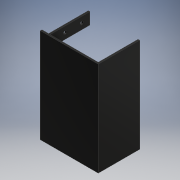
# Autodesk Inventor part: elbow servo plate
Saved by Autodesk Inventor 2017 (Build 210142000, 142)
## iProperties
Created: 2018-10-18
Part Number: elbow servo plate
Material: Generic
Document SubType Name: Modeling
Designer: Cameron
Density: 1 g/cm^3
Appearance: Glossy - Black
Author: Cameron
Autodesk Inventor part; units mm, degrees
ref_plane "YZ Plane" through (0, 0, 0) normal (1, 0, 0) x (0, 1, 0)
ref_plane "XZ Plane" through (0, 0, 0) normal (0, 1, 0) x (-1, 0, 0)
ref_plane "XY Plane" through (0, 0, 0) normal (0, 0, 1) x (1, 0, 0)
sketch "Sketch1" plane through (0, 0, 0) normal (0, 1, 0) x (-1, 0, 0)
  line L0 (0, 0) -> (35, 0)
  line L1 (35, 0) -> (35, -57)
  line L2 (35, -57) -> (0, -57)
  line L3 (0, -57) -> (0, 0)
  dimension "d0" = 35
  dimension "d1" = 57
  constraints: 8 end point, 2 parallel, 1 horizontal, 1 perpendicular
  measures "d0" distance of L1.end L2.end
  measures "d1" distance of L0.end L1.end
extrude "Extrusion1" add sketch "Sketch1" along normal blind 1
sketch "Sketch2" plane through (0, 1, 0) normal (0, 1, 0) x (1, 0, 0)
  line L0 (-35, 0) -> (0, 0) projected
  line L1 (0, 57) -> (-35, 57) projected
  line L2 (0, 0) -> (-1, 0)
  line L3 (-1, 0) -> (-1, 57)
  line L4 (-1, 57) -> (0, 57)
  line L5 (0, 57) -> (0, 0)
  line L6 (-31, 0) -> (-30, 0)
  line L7 (-30, 0) -> (-30, 7)
  line L8 (-30, 7) -> (-31, 7)
  line L9 (-31, 7) -> (-31, 0)
  line L10 (-31, 57) -> (-30, 57)
  line L11 (-30, 57) -> (-30, 50)
  line L12 (-30, 50) -> (-31, 50)
  line L13 (-31, 50) -> (-31, 57)
  dimension "d4" = 1
  dimension "d5" = 31
  dimension "d6" = 1
  dimension "d7" = 7
  dimension "d8" = 7
  constraints: 24 end point, 8 point on line, 5 perpendicular, 2 parallel, 1 horizontal
  measures "d4" distance of L3.end L4.end
  measures "d5" distance of L0.end L6.start
  measures "d6" distance of L6.start L6.end
  measures "d7" distance of L6.end L7.end
  measures "d8" distance of L10.end L11.end
extrude "Extrusion2" add sketch "Sketch2" along normal blind 24
sketch "Sketch3" plane through (-30, 1, 0) normal (1, 0, 0) x (0, 0, -1)
  line L0 (0, 24) -> (7, 24) projected
  line L1 (3.5, 24) -> (3.5, 19)
  line L2 (3.5, 19) -> (3.5, 9)
  line L3 (50, 24) -> (57, 24) projected
  line L4 (53.5, 24) -> (53.5, 19)
  line L5 (53.5, 19) -> (53.5, 9)
  circle A0 centre (3.5, 19) radius 1
  circle A1 centre (3.5, 9) radius 1
  circle A2 centre (53.5, 19) radius 1
  circle A3 centre (53.5, 9) radius 1
  point P0 (0, -1)
  dimension "d11" = 5
  dimension "d12" = 10
  dimension "d13" = 5
  dimension "d14" = 10
  dimension "d15" = 2
  dimension "d16" = 2
  dimension "d17" = 2
  dimension "d18" = 2
  constraints: 8 end point, 4 centre point, 4 coincident, 2 midpoint, 2 point on line, 2 vertical
  measures "d11" distance of L1.start L1.end
  measures "d12" distance of L1.end L2.end
  measures "d13" distance of L4.start L4.end
  measures "d14" distance of L4.end L5.end
  measures "d15" diameter of A0
  measures "d16" diameter of A1
  measures "d17" diameter of A2
  measures "d18" diameter of A3
extrude "Extrusion3" cut sketch "Sketch3" against normal blind 24
body "Solid1"
